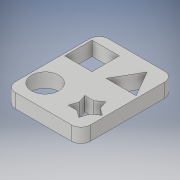
# Autodesk Inventor part: passenger base
Saved by Autodesk Inventor 2018 (Build 220112000, 112)
## iProperties
Created: 2019-01-09
Part Number: passenger base
Material: Generic
Document SubType Name: Modeling
Designer: mimss21
Density: 1 g/cm^3
Appearance: Default
Author: mimss21
Autodesk Inventor part; units mm, degrees
ref_plane "YZ Plane" through (0, 0, 0) normal (1, 0, 0) x (0, 1, 0)
ref_plane "XZ Plane" through (0, 0, 0) normal (0, 1, 0) x (-1, 0, 0)
ref_plane "XY Plane" through (0, 0, 0) normal (0, 0, 1) x (1, 0, 0)
sketch "Sketch1" plane through (0, 0, 0) normal (0, 1, 0) x (-1, 0, 0)
  line L0 (5.08, 0) -> (35.306, 0)
  line L1 (40.386, -5.08) -> (40.386, -45.085)
  line L2 (35.306, -50.165) -> (5.08, -50.165)
  line L3 (0, -45.085) -> (0, -5.08)
  line L4 (1.27, 0) -> (1.27, -50.165) construction
  line L5 (9.3726, 0) -> (9.3726, -50.165) construction
  circle A0 centre (31.75, -12.446) radius 7.366
  line L6 (24.384, -30.353) -> (39.116, -30.353)
  line L7 (39.116, -30.353) -> (39.116, -45.085)
  line L8 (39.116, -45.085) -> (24.384, -45.085)
  line L9 (24.384, -45.085) -> (24.384, -30.353)
  line L10 (9.3726, -45.085) -> (1.27, -31.0388)
  line L11 (1.27, -31.0388) -> (17.4752, -31.0388)
  line L12 (9.3726, -45.085) -> (17.4752, -31.0388)
  circle A1 centre (8.9535, -12.7635) radius 7.6835 construction
  line L13 (15.1696, -17.2797) -> (6.5792, -20.0709) construction
  line L14 (6.5792, -20.0709) -> (1.27, -12.7635) construction
  line L15 (1.27, -12.7635) -> (6.5792, -5.4561) construction
  line L16 (6.5792, -5.4561) -> (15.1696, -8.2473) construction
  line L17 (15.1696, -8.2473) -> (15.1696, -17.2797) construction
  line L18 (15.1696, -17.2797) -> (10.4198, -17.2797)
  line L19 (10.4198, -17.2797) -> (6.5792, -20.0709)
  line L20 (2.1805, -11.5103) -> (8.0524, -19.5923) construction
  line L21 (8.0524, -5.9347) -> (2.1805, -14.0167) construction
  line L22 (5.6687, -6.7092) -> (15.1696, -9.7963) construction
  line L23 (13.6964, -7.7686) -> (13.6964, -17.7584) construction
  line L24 (1.27, -12.7635) -> (5.1164, -15.5513)
  line L25 (5.1164, -15.5513) -> (6.5792, -20.0709)
  line L26 (1.27, -12.7635) -> (5.1164, -9.9757)
  line L27 (5.1164, -9.9757) -> (6.5792, -5.4561)
  line L28 (6.5792, -5.4561) -> (10.4191, -8.2528)
  line L29 (10.4191, -8.2528) -> (15.1696, -8.2473)
  line L30 (15.1696, -8.2473) -> (13.6964, -12.7635)
  line L31 (13.6964, -12.7635) -> (15.1696, -17.2797)
  arc A2 (40.386, -5.08) -> (35.306, 0) centre (35.306, -5.08) ccw
  arc A3 (35.306, -50.165) -> (40.386, -45.085) centre (35.306, -45.085) ccw
  arc A4 (0, -45.085) -> (5.08, -50.165) centre (5.08, -45.085) ccw
  arc A5 (5.08, 0) -> (0, -5.08) centre (5.08, -5.08) ccw
  point P0 (0, 0)
  point P1 (40.386, -50.165)
  point P2 (40.386, 0)
  point P3 (0, -50.165)
  dimension "d0" = 40.386
  dimension "d1" = 50.165
  dimension "d2" = 1.27
  dimension "d3" = 8.1026
  dimension "d4" = 5.08
  dimension "d5" = 14.732
  dimension "d6" = 8.636
  dimension "d7" = 12.446
  dimension "d8" = 1.27
  dimension "d9" = 5.08
  dimension "d10" = 14.732
  dimension "d11" = 14.732
  dimension "d12" = 19.1262
  dimension "d13" = 16.2052
  dimension "d14" = 15.367
  dimension "d15" = 8.9535
  dimension "d16" = 12.7635
  dimension "d17" = 4.7498
  dimension "d18" = 1.4678
  dimension "d19" = 1.4732
  dimension "d20" = 1.4732
  dimension "d21" = 1.4732
  dimension "d22" = 1.4732
  dimension "d23" = 5.08
  constraints: 64 end point, 26 point on line, 11 point on circle, 8 tangent, 6 centre point, 6 parallel, 5 perpendicular, 4 midpoint, 3 equal radius, 3 horizontal, 1 coincident, 1 vertical, 11 other
  measures "d0" distance of point (40.386, -50.165) point (0, -50.165)
  measures "d1" distance of point (40.386, 0) point (40.386, -50.165)
  measures "d2" distance between parallel lines of L3 L4
  measures "d3" distance between parallel lines of L4 L5
  measures "d4" distance from line of L2 L10.start
  measures "d5" diameter of A0
  measures "d6" distance from line of L1 A0.centre
  measures "d7" distance from line of L0 A0.centre
  measures "d8" distance between parallel lines of L1 L7
  measures "d9" distance between parallel lines of L2 L8
  measures "d10" distance of L8.end L6.start
  measures "d11" distance of L6.start L6.end
  measures "d12" distance from line of L2 L10.end
  measures "d13" distance of L10.end L11.end
  measures "d14" diameter of A1
  measures "d15" distance from line of L3 A1.centre
  measures "d16" distance from line of L0 A1.centre
  measures "d17" distance of L13.start L18.end
  measures "d18" distance from line of L13 L18.end
  measures "d19" distance between parallel lines of L14 L20
  measures "d20" distance between parallel lines of L17 L23
  measures "d21" distance between parallel lines of L16 L22
  measures "d22" distance between parallel lines of L15 L21
  measures "d23" radius of A2
extrude "Extrusion1" add sketch "Sketch1" along normal blind 7.62
shell "Shell1" thickness 0.254 removed faces 1 at (-17.0773, 0, -40.4029)
body "Solid1"
